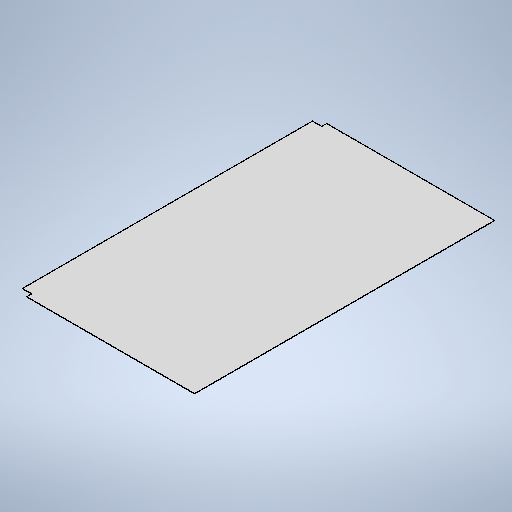
# Autodesk Inventor part: GnG frame 2 floor sheet 6
Saved by Autodesk Inventor 2025.3 (Build 293356000, 356)
## iProperties
Created: 2025-10-28
Part Number: GnG frame 2 floor sheet 6
Material: Stainless Steel
Document SubType Name: Sheet Metal
Designer: admin
Mass: 280.619 g
Surface Area: 364.406 cm^2
Volume: 35.0774 cm^3
Density: 8 g/cm^3
Sheet Metal Rule: AISI304 3mm Die 32
Sheet Metal Width: 1240,000 mm
Sheet Metal Length: 2100,000 mm
Sheet Metal Area: 2604000,000 mm^2
Appearance: Default
Flat Pattern Width: 124 cm
Flat Pattern Length: 210 cm
Flat Pattern Area: 26040 cm^2
Author: admin
Autodesk Inventor part; units mm, degrees
ref_plane "YZ Plane" through (0, 0, 0) normal (1, 0, 0) x (0, 1, 0)
ref_plane "XZ Plane" through (0, 0, 0) normal (0, 1, 0) x (-1, 0, 0)
ref_plane "XY Plane" through (0, 0, 0) normal (0, 0, 1) x (1, 0, 0)
sketch "Sketch1" plane through (0, 0, 0) normal (0, 0, 1) x (1, 0, 0)
  line L0 (0, 0) -> (-1240, 0)
  line L1 (-1240, 0) -> (-1240, -2100)
  line L2 (-1240, -2100) -> (0, -2100)
  line L3 (0, -2100) -> (0, 0)
  line L4 (0, 0) -> (-65, 0)
  line L5 (-65, 0) -> (-65, -35)
  line L6 (-65, -35) -> (0, -35)
  line L7 (0, -35) -> (0, 0)
  line L8 (0, -2100) -> (-65, -2100)
  line L9 (-65, -2100) -> (-65, -2065)
  line L10 (-65, -2065) -> (0, -2065)
  line L11 (0, -2065) -> (0, -2100)
  line L12 (-1240, 0) -> (-1175, 0)
  line L13 (-1175, 0) -> (-1175, -35)
  line L14 (-1175, -35) -> (-1240, -35)
  line L15 (-1240, -35) -> (-1240, 0)
  line L16 (-1240, -2100) -> (-1175, -2100)
  line L17 (-1175, -2100) -> (-1175, -2065)
  line L18 (-1175, -2065) -> (-1240, -2065)
  line L19 (-1240, -2065) -> (-1240, -2100)
  line L20 (-1125, -2100) -> (-1035, -2100)
  line L21 (-1035, -2100) -> (-1035, -2065)
  line L22 (-1035, -2065) -> (-1125, -2065)
  line L23 (-1125, -2065) -> (-1125, -2100)
  line L24 (-1125, 0) -> (-1035, 0)
  line L25 (-1035, 0) -> (-1035, -35)
  line L26 (-1035, -35) -> (-1125, -35)
  line L27 (-1125, -35) -> (-1125, 0)
  point P0 (0, -35)
  point P1 (-65, 0)
  point P2 (-65, -2100)
  point P3 (0, -2065)
  point P4 (-1035, -2100)
  point P5 (-1035, 0)
  point P6 (-1175, 0)
  point P7 (-1175, -2100)
  dimension "d22" = 1240
  dimension "d23" = 2100
  dimension "d24" = 65
  dimension "d25" = 35
  dimension "d28" = 90
  dimension "d29" = 970
  measures "d22" distance of L2.end L1.end
  measures "d23" distance of L1.end L0.end
  measures "d24" distance of L6.end L5.end
  measures "d25" distance of L5.end L4.end
  measures "d28" distance of L25.end L26.end
  measures "d29" distance between parallel lines of L5 L25
extrude "Plate1" add sketch "Sketch1" along normal blind 3 contours L3 L6 L5 L0 | L5 L6 L3 L10 L9 L2 L21 L22 L23 L17 L18 L1 L14 L13 L0 L27 L26 L25 | L25 L26 L27 L0 | L3 L2 L9 L10 | L2 L23 L22 L21
sketch "Sketch5" plane through (0, 0, 0) normal (0, 0, -1) x (-1, 0, 0)
  line L0 (1175, 0) -> (1075, 0) construction
  line L1 (1075, 0) -> (1075, -2) construction
  line L2 (1075, -2) -> (1175, -2) construction
  line L3 (1175, -2) -> (1175, 0) construction
  line L4 (1075, 0) -> (1073.4752, -4.6556)
  arc A0 (1072.5248, -4.6556) -> (1073.4752, -4.6556) centre (1073, -4.5) ccw
  line L5 (1072.5248, -4.6556) -> (1071, 0)
  line L6 (1071, 0) -> (1075, 0)
  line L7 (1071, 0) -> (1069, 0) construction
  line L8 (1069, 0) -> (1067, 0)
  line L9 (1067, 0) -> (1067, -5)
  line L10 (1067, -5) -> (1069, -5)
  line L11 (1069, -5) -> (1069, 0)
  line L12 (1067, 0) -> (1065, 0) construction
  line L13 (1065, 0) -> (1063, 0)
  line L14 (1063, 0) -> (1063, -5)
  line L15 (1063, -5) -> (1065, -5)
  line L16 (1065, -5) -> (1065, 0)
  line L17 (1063, 0) -> (1061, 0) construction
  line L18 (1061, 0) -> (1059, 0)
  line L19 (1059, 0) -> (1059, -5)
  line L20 (1059, -5) -> (1061, -5)
  line L21 (1061, -5) -> (1061, 0)
  line L22 (1059, 0) -> (1057, 0) construction
  line L23 (1057, 0) -> (1055, 0)
  line L24 (1055, 0) -> (1055, -5)
  line L25 (1055, -5) -> (1057, -5)
  line L26 (1057, -5) -> (1057, 0)
  line L27 (1055, 0) -> (1050, 0) construction
  line L28 (1050, 0) -> (1045, 0) construction
  circle A1 centre (1050, 0) radius 1
  circle A2 centre (1045, 0) radius 1
  line L29 (0, 0) -> (1175, 0) projected
  point P0 (1175, 0)
  point P1 (1073, 0)
  dimension "d30" = 100
  dimension "d31" = 2
  dimension "d32" = 5
  dimension "d33" = 4
  dimension "d34" = 0.5
  dimension "d35" = 5
  dimension "d36" = 5
  dimension "d37" = 5
  dimension "d38" = 2
  constraints: 58 end point, 11 horizontal, 10 equal length, 10 parallel, 5 perpendicular, 3 centre point, 3 coincident, 3 tangent, 2 point on circle, 1 equal radius, 1 midpoint, 1 point on line, 1 vertical alignment
  measures "d30" distance of L2.end L1.end
  measures "d31" distance of L1.end L0.end
  measures "d32" distance of L9.end L9.start
  measures "d33" distance of L5.end L0.end
  measures "d34" radius of A0
  measures "d35" distance of L15.start L13.end
  measures "d36" distance of L19.end L19.start
  measures "d37" distance of L24.end L24.start
  measures "d38" diameter of A1
extrude "Cut1" cut sketch "Sketch5" against normal blind 3 contours A2 L29 | L29 A2 | A1 L29 | L29 A1 | L26 L25 L24 L23 | L21 L20 L19 L18
equation "\"d33\" = 2 * d31"
equation "\"d34\" = 0.25 * d31"
equation "\"d38\" = d31"
equation "\"d39\" = Thickness"
equation "\"d2\" = Thickness"
equation "\"BendReliefWidth\" = Thickness"
equation "\"BendReliefDepth\" = 0.5 * Thickness"
equation "\"CornerReliefSize\" = 4 * Thickness"
equation "\"MinimumRemnant\" = 2 * Thickness"
equation "\"TransitionRadius\" = BendRadius"
equation "\"JacobiRadiusSize\" = BendRadius"
equation "\"GapSize\" = Thickness"
equation "\"Thickness\" = 3"
equation "\"BendRadius\" = 5"
body "Solid1"
